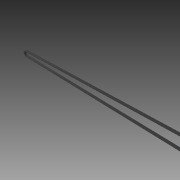
# Autodesk Inventor part: y_axis_belt
Saved by Autodesk Inventor 2014 (Build 180170000, 170)
## iProperties
Created: 2014-03-26
Part Number: y_axis_belt
Material: Rubber
Document SubType Name: Modeling
Designer: buben
Density: 0.93 g/cm^3
Appearance: Rubber - Black - Version 1.1
Author: buben
Autodesk Inventor part; units mm, degrees
ref_plane "YZ Plane" through (0, 0, 0) normal (1, 0, 0) x (0, 1, 0)
ref_plane "XZ Plane" through (0, 0, 0) normal (0, 1, 0) x (-1, 0, 0)
ref_plane "XY Plane" through (0, 0, 0) normal (0, 0, 1) x (1, 0, 0)
sketch "Sketch1" plane through (0, 0, 0) normal (0, 1, 0) x (-1, 0, 0)
  line L0 (0.1032, -6.0991) -> (-407.6831, -12.9981)
  line L1 (0.1032, 6.0991) -> (-407.6831, 12.9981)
  arc A0 (0.1032, -6.0991) -> (0.1032, 6.0991) centre (0, 0) ccw
  arc A1 (-407.6831, 12.9981) -> (-407.6831, -12.9981) centre (-407.903, 0) ccw
  line L2 (-407.6598, 14.3779) -> (0.1265, 7.4789)
  arc A2 (0.1265, -7.4789) -> (0.1265, 7.4789) centre (0, 0) ccw
  line L3 (0.1265, -7.4789) -> (-407.6598, -14.3779)
  arc A3 (-407.6598, 14.3779) -> (-407.6598, -14.3779) centre (-407.903, 0) ccw
  dimension "d2" = 6.1
  dimension "d3" = 13
  dimension "d4" = 1.38
  dimension "d5" = 407.903
  constraints: 8 end point, 8 point on circle, 4 centre point, 4 tangent, 1 coincident, 1 horizontal alignment, 3 other
  measures "d2" radius of A0
  measures "d3" radius of A1
  measures "d4" distance between parallel lines of L2 L1
  measures "d5" distance of A1.centre point (0, 0)
extrude "Extrusion1" add sketch "Sketch1" along normal blind 6
chamfer "Chamfer1" distance 0.2 angle 45 16 edges at (203.79, 6, 9.5486) (-6.1, 6, 0) (203.79, 6, -9.5486) (420.903, 6, 0) (203.7666, 6, 10.9284) (422.283, 6, 0) (203.7666, 6, -10.9284) (-7.48, 6, 0) (203.7666, 0, 10.9284) (-7.48, 0, 0) (203.7666, 0, -10.9284) (422.283, 0, 0) (203.79, 0, 9.5486) (420.903, 0, 0) (203.79, 0, -9.5486) (-6.1, 0, 0)
body "Solid1"
